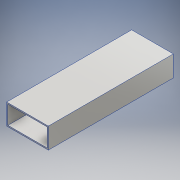
# Autodesk Inventor part: tube
Saved by Autodesk Inventor 2016 (Build 200138000, 138)
## iProperties
Created: 2016-07-19
Part Number: tube
Material: Aluminum 6061
Document SubType Name: Modeling
Designer: Jonathan
Density: 2.7 g/cm^3
Appearance: Aluminum - Flat
Author: Jonathan
Autodesk Inventor part; units mm, degrees
ref_plane "YZ Plane" through (0, 0, 0) normal (1, 0, 0) x (0, 1, 0)
ref_plane "XZ Plane" through (0, 0, 0) normal (0, 1, 0) x (-1, 0, 0)
ref_plane "XY Plane" through (0, 0, 0) normal (0, 0, 1) x (1, 0, 0)
sketch "Sketch1" plane through (0, 0, 0) normal (0, 1, 0) x (-1, 0, 0)
  line L0 (50.8, 25.4) -> (-50.8, 25.4)
  line L1 (-50.8, 25.4) -> (-50.8, -25.4)
  line L2 (-50.8, -25.4) -> (50.8, -25.4)
  line L3 (50.8, -25.4) -> (50.8, 25.4)
  line L4 (-47.625, 22.225) -> (47.625, 22.225)
  line L5 (47.625, 22.225) -> (47.625, -22.225)
  line L6 (47.625, -22.225) -> (-47.625, -22.225)
  line L7 (-47.625, -22.225) -> (-47.625, 22.225)
  point P0 (0, 0)
  point P1 (50.8, 0)
  point P2 (0, 25.4)
  dimension "d0" = 50.8
  dimension "d1" = 101.6
  dimension "d7" = 3.175
  constraints: 16 end point, 4 parallel, 2 midpoint, 2 perpendicular, 1 horizontal, 1 horizontal alignment, 1 vertical alignment, 3 other
  measures "d0" distance of L2.end L0.start
  measures "d1" distance of L1.end L2.end
  measures "d7" distance between parallel lines of L0 L4
extrude "Extrusion1" add sketch "Sketch1" along normal blind 304.8
body "Solid1"
